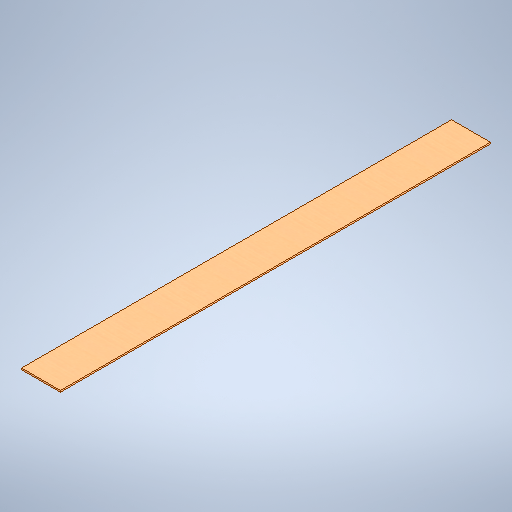
# Autodesk Inventor part: Base_Entera
Saved by Autodesk Inventor 2025.2 (Build 292293000, 293)
## iProperties
Created: 2025-05-13
Part Number: Base_Entera
Material: Wood (Cherry)
Document SubType Name: Modeling
Designer: USER
Density: 0.63 g/cm^3
Appearance: Cherry - Natural Low Gloss
Author: USER
Autodesk Inventor part; units mm, degrees
ref_plane "YZ Plane" through (0, 0, 0) normal (1, 0, 0) x (0, 1, 0)
ref_plane "XZ Plane" through (0, 0, 0) normal (0, 1, 0) x (-1, 0, 0)
ref_plane "XY Plane" through (0, 0, 0) normal (0, 0, 1) x (1, 0, 0)
sketch "Sketch1" plane through (0, 0, 0) normal (0, 1, 0) x (-1, 0, 0)
  line L0 (0, 0) -> (150, 0)
  line L1 (150, 0) -> (150, -1660)
  line L2 (150, -1660) -> (0, -1660)
  line L3 (0, -1660) -> (0, 0)
  dimension "d0" = 150
  dimension "d1" = 1660
  constraints: 8 end point, 2 parallel, 1 horizontal, 1 perpendicular
  measures "d0" distance of L1.end L2.end
  measures "d1" distance of L0.end L1.end
extrude "Extrusion1" add sketch "Sketch1" along normal blind 6
move faces "Move1" translate (0, 0, 53) faces at (-50, 2, -1660)
move faces "Move2" translate (0, 0, 53) faces at (-50, 4, 0)
body "Solid1"
